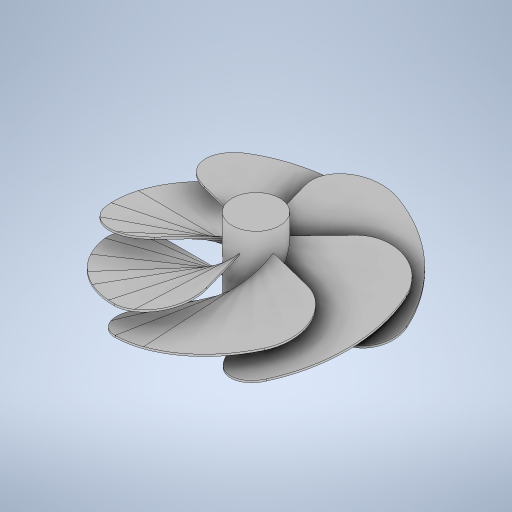
# Autodesk Inventor part: Hélice
Saved by Autodesk Inventor 2023 (Build 270158030, 158C)
## iProperties
Created: 2022-06-22
Part Number: Hélice
Material: Genérico
Document SubType Name: Modeling
Designer: robofei
Density: 1 g/cm^3
Appearance: Padrão
Author: robofei
Autodesk Inventor part; units mm, degrees
ref_plane "YZ Plane" through (0, 0, 0) normal (1, 0, 0) x (0, 1, 0)
ref_plane "XZ Plane" through (0, 0, 0) normal (0, 1, 0) x (-1, 0, 0)
ref_plane "XY Plane" through (0, 0, 0) normal (0, 0, 1) x (1, 0, 0)
sketch "Sketch1" plane through (0, 0, 0) normal (0, 1, 0) x (-1, 0, 0)
  circle A0 centre (0, 0) radius 25
  dimension "d0" = 50
  constraints: 1 centre point, 1 coincident
  measures "d0" diameter of A0
extrude "Extrusion1" add sketch "Sketch1" along normal blind 80
sketch "Sketch2" plane through (0, 0, 0) normal (0, 0, 1) x (1, 0, 0)
  line L0 (-125, 6) -> (-25, 6)
  line L1 (-25, 6) -> (-25, 8)
  line L2 (-25, 8) -> (-125, 8)
  line L3 (-125, 8) -> (-125, 6)
  line L4 (0, -9.5812) -> (0, 97.6007) construction
  line L5 (25, 0) -> (-25, 0) projected
  point P0 (0, 0)
  dimension "d3" = 100
  dimension "d4" = 2
  dimension "d6" = 6
  dimension "d8" = 25
  constraints: 10 end point, 2 parallel, 2 vertical, 1 horizontal, 1 perpendicular
  measures "d3" distance of L2.end L1.end
  measures "d4" distance of L1.end L0.end
  measures "d6" distance between parallel lines of L5 L0
  measures "d8" distance from line of L4 L0.end
coil "Coil1" sketch "Sketch2" operation add axis through (0, -9.5812, 0) along (0, 1, 0) pitch 170 turns 0.294118 hand right
fillet "Fillet1" radius 30 1 edges at (-125, 7, 0)
fillet "Fillet2" radius 40 1 edges at (34.2079, 57, 120.2282)
pattern_circular "Circular Pattern1" count 6 over 360 about axis through (0, 0, 0) along (0, 1, 0) of "Fillet2", "Fillet1", "Coil1"
body "Solid1"
